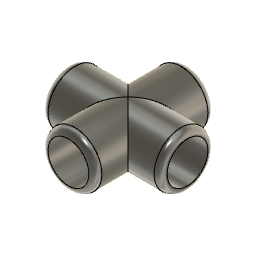
Connector_-_X_shaped (Autodesk Fusion 360 design; units mm, degrees)
Autodesk Fusion 360 part; units mm, degrees
cylinder "CylinderPrimitive1" add diameter 16.5 height 36.5 placed x (1, 0, 0) y (0, 1, 0) z (0, 0, 1) at (0, 0, 0) makes body 1
cylinder "CylinderPrimitive2" add diameter 16.5 height 36.5 placed x (1, 0, 0) y (0, 0, -1) z (0, 1, 0) at (30, 0, 0) separate body makes body 2
cylinder "CylinderPrimitive3" cut diameter 12.5 height -44 placed x (1, 0, 0) y (0, 0, 1) z (0, -1, 0) at (30, 0, 0) bodies 2
cylinder "CylinderPrimitive4" cut diameter 12.5 height 44 placed x (1, 0, 0) y (0, 1, 0) z (0, 0, 1) at (0, 0, 0) bodies 1
move_body "Move1" bodies 2 to x (1, 0, 0) y (0, 1, 0) z (0, 0, 1) at (-30, -18.25, 18.25)
combine "Combine1" operation add target body 1 tool bodies 2
cylinder "CylinderPrimitive5" cut diameter 12.5 height -44 placed x (1, 0, 0) y (0, 1, 0) z (0, 0, 1) at (0, 0, 36.5) bodies 1
cylinder "CylinderPrimitive6" cut diameter 12.5 height -44 placed x (1, 0, 0) y (0, 0, -1) z (0, 1, 0) at (0, 18.25, 18.25) bodies 1
fillet "Fillet1" radius 2 4 edges at (-7.6917, -2.9833, 36.5) (-7.6917, 18.25, 21.2333) (-7.6917, -18.25, 15.2667) (-7.6917, 2.9833, 0) on bodies 1
move_body "Move2" bodies 1 to x (0, 0, -1) y (0, 1, 0) z (1, 0, 0) at (-8.25, 0, -8.25)
move_body "Move3" bodies 1 to x (1, 0, 0) y (0, 1, 0) z (0, 0, 1) at (-10, 0, 0)
move_body "Move4" bodies 1 to x (1, 0, 0) y (0, 1, 0) z (0, 0, 1) at (0, 0, 16.5)
